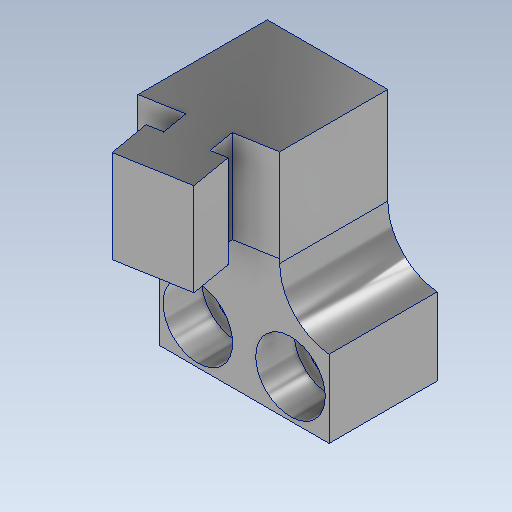
# Autodesk Inventor part: Finray_9_Kerbe_10deg_anschluss_erweitert_9_75 Nut
Saved by Autodesk Inventor 2025.2 (Build 292293000, 293)
## iProperties
Created: 2022-02-28
Part Number: Finray_9_Kerbe_10deg_anschluss_erweitert_9_75 Nut
Material: Generic
Document SubType Name: Modeling
Designer: richa
Density: 1 g/cm^3
Appearance: Aluminum - Flat
Author: richa
Autodesk Inventor part; units mm, degrees
ref_plane "YZ Plane" through (0, 0, 0) normal (1, 0, 0) x (0, 1, 0)
ref_plane "XZ Plane" through (0, 0, 0) normal (0, 1, 0) x (-1, 0, 0)
ref_plane "XY Plane" through (0, 0, 0) normal (0, 0, 1) x (1, 0, 0)
sketch "Sketch5" plane through (0, 0, 0) normal (0, 0, 1) x (1, 0, 0)
  line L0 (0, 0) -> (-15.6, 0)
  line L1 (-15.6, 0) -> (-15.6, -29.5)
  line L2 (-15.6, -29.5) -> (6.4, -29.5)
  line L3 (6.4, -29.5) -> (6.4, -19.5)
  line L4 (0, 0) -> (0, -12.526)
  line L5 (0, -12.526) -> (0, -19.5)
  line L6 (0, -19.5) -> (6.4, -19.5)
  dimension "d111" = 15.6
  dimension "d112" = 29.5
  dimension "d113" = 22
  dimension "d114" = 10
  dimension "d116" = 12.526
  constraints: 14 end point, 4 perpendicular, 2 vertical, 1 horizontal
  measures "d111" distance of L0.start L0.end
  measures "d112" distance of L0.end L1.end
  measures "d113" distance of L1.end L2.end
  measures "d114" distance of L2.end L3.end
  measures "d116" distance of L0.start L4.end
extrude "Extrusion2" add sketch "Sketch5" along normal blind 14
sketch "Skizze14" plane through (0, 0, 14) normal (0, 0, 1) x (1, 0, 0)
  line L0 (-15.6, -29.5) -> (6.4, -29.5) projected
  line L1 (-15.6, 0) -> (-15.6, -29.5) projected
  circle A0 centre (-10.6, -24.5) radius 4.5
  circle A1 centre (1.4, -24.5) radius 4.5
  circle A2 centre (-10.6, -24.5) radius 2.75
  circle A3 centre (1.4, -24.5) radius 2.75
  point P0 (0, 0)
  dimension "d117" = 5
  dimension "d118" = 5
  dimension "d119" = 12
  dimension "d120" = 5
  dimension "d121" = 9
  dimension "d122" = 9
  dimension "d123" = 5.5
  dimension "d124" = 5.5
  constraints: 4 centre point, 4 coincident
  measures "d117" distance from line of L0 point (-10.6, -24.5)
  measures "d118" distance from line of L1 point (-10.6, -24.5)
  measures "d119" distance of point (1.4, -24.5) point (-10.6, -24.5)
  measures "d120" distance from line of L0 point (1.4, -24.5)
  measures "d121" diameter of A0
  measures "d122" diameter of A1
  measures "d123" diameter of A2
  measures "d124" diameter of A3
extrude "Extrusion9" cut sketch "Skizze14" against normal blind 5 contours A0 | A1 | A2 | A3
sketch "Skizze16" plane through (0, 0, 14) normal (0, 0, 1) x (1, 0, 0)
  circle A0 centre (-10.6, -24.5) radius 2.75
  circle A1 centre (1.4, -24.5) radius 2.75
  line L0 (-15.6, 0) -> (-15.6, -29.5) projected
  line L1 (-15.6, -29.5) -> (6.4, -29.5) projected
  line L2 (6.4, -29.5) -> (6.4, -19.5) projected
  point P0 (0, 0)
  dimension "d127" = 5
  dimension "d128" = 5
  dimension "d129" = 5
  dimension "d130" = 5
  dimension "d131" = 5.5
  dimension "d132" = 5.5
  constraints: 2 centre point
  measures "d127" distance from line of L0 A0.centre
  measures "d128" distance from line of L1 A0.centre
  measures "d129" distance from line of L1 A1.centre
  measures "d130" distance from line of L2 A1.centre
  measures "d131" diameter of A0
  measures "d132" diameter of A1
extrude "Extrusion10" cut sketch "Skizze16" against normal blind 15
fillet "Rundung3" radius 7 1 edges at (0, -19.5, 7)
sketch "Skizze17" plane through (-15.6, 0, 0) normal (0, 1, 0) x (1, 0, 0)
  line L0 (0, -14) -> (22, -14) projected
  line L1 (0, -14) -> (0, -16.751)
  line L2 (0, -16.751) -> (5.264, -15.8228)
  line L3 (5.8718, -19.2696) -> (3.9022, -19.6169)
  line L4 (3.9022, -19.6169) -> (4.8399, -24.9349)
  line L5 (4.8399, -24.9349) -> (13.8508, -23.346)
  line L6 (10.3562, -14.9105) -> (15.6, -14)
  line L7 (5.264, -15.8228) -> (5.8718, -19.2696)
  line L8 (13.8508, -23.346) -> (12.9251, -18.0147)
  line L9 (12.9251, -18.0147) -> (10.9546, -18.3569)
  line L10 (10.9546, -18.3569) -> (10.3562, -14.9105)
  point P0 (15.6, 0)
  dimension "d136" = 2.751
  dimension "d137" = 80
  dimension "d141" = 3.5
  dimension "d143" = 2
  dimension "d144" = 5.4
  dimension "d145" = 9.15
  dimension "d147" = 2
  constraints: 20 end point, 2 perpendicular, 1 point on line, 1 vertical
  measures "d136" distance of L0.start L1.end
  measures "d137" angle of L2 L1
  measures "d141" distance of L2.end L3.start
  measures "d143" distance of L3.start L3.end
  measures "d144" distance of L3.end L4.end
  measures "d145" distance of L4.end L5.end
  measures "d147" distance of L8.end L9.end
extrude "Extrusion11" add sketch "Skizze17" against normal blind 12
equation "\"l1\" = 8"
body "Solid2"
